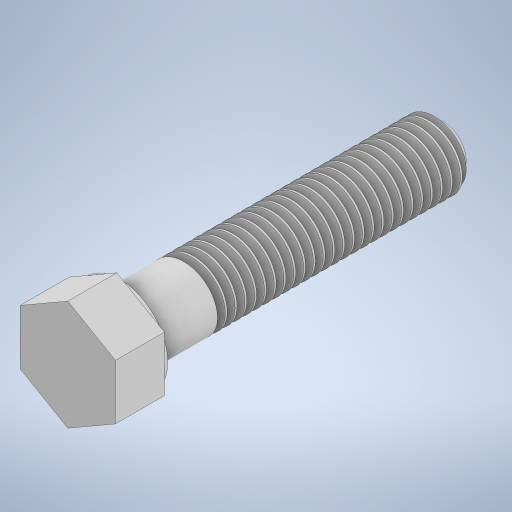
# Autodesk Inventor part: Parafuso
Saved by Autodesk Inventor 2023 (Build 270158030, 158C)
## iProperties
Created: 2022-07-20
Part Number: Parafuso
Material: Generic
Document SubType Name: Modeling
Designer: coqui
Density: 1 g/cm^3
Appearance: Default
Author: coqui
Autodesk Inventor part; units mm, degrees
ref_plane "YZ Plane" through (0, 0, 0) normal (1, 0, 0) x (0, 1, 0)
ref_plane "XZ Plane" through (0, 0, 0) normal (0, 1, 0) x (-1, 0, 0)
ref_plane "XY Plane" through (0, 0, 0) normal (0, 0, 1) x (1, 0, 0)
sketch "Sketch1" plane through (0, 0, 0) normal (0, 0, 1) x (1, 0, 0)
  circle A0 centre (0, 0) radius 10
  dimension "d0" = 20
  constraints: 1 centre point, 1 coincident
  measures "d0" diameter of A0
extrude "Extrusion1" add sketch "Sketch1" along normal blind 100
sketch "Sketch2" plane through (0, 0, 100) normal (0, 0, 1) x (1, 0, 0)
  line L0 (0, -16.8462) -> (-14.5892, -8.4231)
  line L1 (-14.5892, -8.4231) -> (-14.5892, 8.4231)
  line L2 (-14.5892, 8.4231) -> (0, 16.8462)
  line L3 (0, 16.8462) -> (14.5892, 8.4231)
  line L4 (14.5892, 8.4231) -> (14.5892, -8.4231)
  line L5 (14.5892, -8.4231) -> (0, -16.8462)
  point P0 (0, 0)
  point P1 (0, 0)
  constraints: 12 end point, 1 coincident, 13 other
extrude "Extrusion2" add sketch "Sketch2" along normal blind 15
chamfer "Chamfer1" distance 3 angle 45 1 edges at (-10, 0, 0)
sketch "Sketch4" plane through (0, 0, 0) normal (0, 1, 0) x (-1, 0, 0)
  line L0 (0, -23.4183) -> (0, 112.0375) construction
  line L1 (78.1703, 0) -> (-105.1553, 0) construction
  line L2 (-11.035, 1.7927) -> (-7.93, 0)
  line L3 (-7.93, 0) -> (-11.035, -1.7927)
  line L4 (-11.035, -1.7927) -> (-11.035, 1.7927)
  point P0 (0, 0)
  point P1 (-10, 0)
  dimension "d10" = 2.07
  dimension "d11" = 10
  dimension "d12" = 0
  constraints: 10 end point, 2 horizontal, 2 vertical, 1 parallel, 7 other
  measures "d10" distance of L2.end point (-10, 0)
  measures "d11" distance from line of L0 point (-10, 0)
  measures "d12" distance from line of L1 point (-10, 0)
coil "Coil1" sketch "Sketch4" operation cut axis through (0, 0, -23.4183) along (0, 0, 1) pitch 3 turns 26.666667 hand right
sketch "Sketch5" plane through (0, 0, 100) normal (0, 0, -1) x (-1, 0, 0)
  circle A0 centre (0, 0) radius 14.5892
  line L0 (14.5892, 8.4231) -> (14.5892, -8.4231) projected
  constraints: 1 centre point, 1 coincident, 1 tangent
extrude "Extrusion4" add sketch "Sketch5" along normal blind 1
sketch "Sketch6" plane through (-5, -8.6603, 78.8049) normal (-0.866, 0.5, 0) x (0, 0, 1)
  line L0 (2.3902, 0) -> (0, 0) projected
  line L1 (1.1951, 2.07) -> (2.3902, 0) projected
  line L2 (0, 0) -> (1.1951, 2.07) projected
  line L3 (2.3902, 0) -> (0, 0) projected
  line L4 (1.1951, 2.07) -> (2.3902, 0) projected
  line L5 (0, 0) -> (1.1951, 2.07) projected
  point P0 (-78.8049, 10)
extrude "Extrusion5" cut sketch "Sketch6" against normal blind 10000
body "Solid1"
